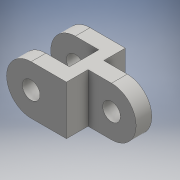
# Autodesk Inventor part: 6_16_V
Saved by Autodesk Inventor 2016 (Build 200138000, 138)
## iProperties
Created: 2016-07-20
Part Number: 6_16_V
Material: Generic
Document SubType Name: Modeling
Designer: cfkguest
Density: 1 g/cm^3
Appearance: Default
Author: cfkguest
Autodesk Inventor part; units mm, degrees
ref_plane "YZ Plane" through (0, 0, 0) normal (1, 0, 0) x (0, 1, 0)
ref_plane "XZ Plane" through (0, 0, 0) normal (0, 1, 0) x (-1, 0, 0)
ref_plane "XY Plane" through (0, 0, 0) normal (0, 0, 1) x (1, 0, 0)
sketch "Sketch1" plane through (0, 0, 0) normal (0, 0, 1) x (1, 0, 0)
  line L0 (-66.3717, -23.5619) -> (-5.3717, -23.5619)
  line L1 (-5.3717, -23.5619) -> (-5.3717, -1.5619)
  line L2 (-5.3717, -1.5619) -> (43.6283, -1.5619)
  line L3 (43.6283, -1.5619) -> (43.6283, 14.4381)
  line L4 (43.6283, 14.4381) -> (-5.3717, 14.4381)
  line L5 (-5.3717, 14.4381) -> (-5.3717, 36.4381)
  line L6 (-5.3717, 36.4381) -> (-66.3717, 36.4381)
  line L7 (-66.3717, 36.4381) -> (-66.3717, 21.4381)
  line L8 (-66.3717, 21.4381) -> (-17.3717, 21.4381)
  line L9 (-17.3717, 21.4381) -> (-17.3717, -8.5619)
  line L10 (-17.3717, -8.5619) -> (-66.3717, -8.5619)
  line L11 (-66.3717, -8.5619) -> (-66.3717, -23.5619)
  point P0 (0, 0)
  dimension "d0" = 15
  dimension "d1" = 15
  dimension "d2" = 60
  dimension "d3" = 12
  dimension "d4" = 61
  dimension "d5" = 22
  dimension "d6" = 22
  dimension "d7" = 49
  dimension "d8" = 43.6283
  dimension "d9" = 1.5619
  constraints: 24 end point, 10 perpendicular, 3 point on line, 1 horizontal
  measures "d0" distance of L6.end L7.end
  measures "d1" distance of L10.end L0.start
  measures "d2" distance between parallel lines of L0 L6
  measures "d3" distance between parallel lines of L9 L5
  measures "d4" distance of L5.end L6.end
  measures "d5" distance of L4.end L5.end
  measures "d6" distance of L0.end L1.end
  measures "d7" distance of L1.end L2.end
  measures "d8" distance from line of point (0, 0) L3
  measures "d9" distance from line of point (0, 0) L2
extrude "Extrusion1" add sketch "Sketch1" along normal blind 50
fillet "Fillet1" radius 25 6 edges at (43.6283, 6.4381, 50) (43.6283, 6.4381, 0) (-66.3717, 28.9381, 50) (-66.3717, -16.0619, 50) (-66.3717, 28.9381, 0) (-66.3717, -16.0619, 0)
sketch "Sketch2" plane through (-5.3717, -23.5619, 0) normal (0, -1, 0) x (1, 0, 0)
  arc A0 (-36, 50) -> (-36, 0) centre (-36, 25) ccw projected
  arc A1 (24, 0) -> (24, 50) centre (24, 25) ccw projected
  point P0 (5.3717, 0)
  constraints: 2 coincident
hole "Hole1" at (-41.3717, -23.5619, 25) at (18.6283, -23.5619, 25) direction (0, 1, 0) diameter 18 end through all
body "Solid1"
